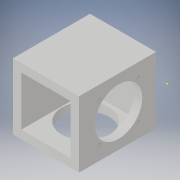
# Autodesk Inventor part: chamber
Saved by Autodesk Inventor 2019 (Build 230136000, 136)
## iProperties
Created: 2019-01-15
Part Number: chamber
Material: Generic
Document SubType Name: Sheet Metal
Designer: voras
Density: 1 g/cm^3
Appearance: Default
Sheet Metal Rule: Default
Author: voras
Autodesk Inventor part; units mm, degrees
ref_plane "YZ Plane" through (0, 0, 0) normal (1, 0, 0) x (0, 1, 0)
ref_plane "XZ Plane" through (0, 0, 0) normal (0, 1, 0) x (-1, 0, 0)
ref_plane "XY Plane" through (0, 0, 0) normal (0, 0, 1) x (1, 0, 0)
sketch "Sketch1" plane through (0, 0, 0) normal (0, 0, 1) x (1, 0, 0)
  point P0 (0, 0)
sketch "Sketch2" plane through (0, 0, 0) normal (0, 0, 1) x (1, 0, 0)
  line L0 (-22.5, 22.5) -> (22.5, 22.5)
  line L1 (22.5, 22.5) -> (22.5, -22.5)
  line L2 (22.5, -22.5) -> (-22.5, -22.5)
  line L3 (-22.5, -22.5) -> (-22.5, 22.5)
  line L4 (-22.5, 22.5) -> (22.5, -22.5) construction
  line L5 (22.5, 22.5) -> (-22.5, -22.5) construction
  line L6 (30, -30) -> (-30, -30)
  line L7 (-30, -30) -> (-30, 30)
  line L8 (-30, 30) -> (30, 30)
  line L9 (30, 30) -> (30, -30)
  line L10 (30, -30) -> (-30, 30) construction
  line L11 (-30, -30) -> (30, 30) construction
  point P0 (0, 0)
  dimension "d0" = 45
  dimension "d1" = 45
  dimension "d2" = 60
  dimension "d3" = 60
  constraints: 24 end point, 4 midpoint, 4 parallel, 2 horizontal, 2 perpendicular
  measures "d0" distance of L1.end L2.end
  measures "d1" distance of L0.end L1.end
  measures "d2" distance of L7.end L8.end
  measures "d3" distance of L6.end L7.end
extrude "Extrusion1" add sketch "Sketch2" along normal blind 55
sketch "Sketch3" plane through (0, 0, 0) normal (0, 0, 1) x (1, 0, 0)
  line L0 (-22.5, 22.5) -> (22.5, 22.5) projected
  line L1 (22.5, 22.5) -> (22.5, -22.5) projected
  line L2 (-22.5, 22.5) -> (22.5, 22.5)
  line L3 (22.5, 22.5) -> (22.5, -22.5)
  line L4 (22.5, -22.5) -> (-22.5, -22.5)
  line L5 (-22.5, -22.5) -> (-22.5, 22.5)
  point P0 (0, 0)
  constraints: 8 end point, 2 parallel, 1 horizontal, 1 perpendicular
extrude "Extrusion2" add sketch "Sketch3" along normal blind 20
sketch "Sketch6" plane through (30, -38.0357, 69.5741) normal (1, 0, 0) x (0, 0, -1)
  circle A0 centre (25.5741, 38.0357) radius 21.5
  line L0 (69.5741, 8.0357) -> (14.5741, 8.0357) projected
  line L1 (14.5741, 8.0357) -> (14.5741, 68.0357) projected
  point P0 (30, 0)
  dimension "d36" = 43
  dimension "d37" = 30
  dimension "d38" = 11
  constraints: 1 centre point
  measures "d36" diameter of A0
  measures "d37" distance from line of L0 A0.centre
  measures "d38" distance from line of A0.centre L1
extrude "Extrusion5" cut sketch "Sketch6" against normal blind 20
sketch "Sketch5" plane through (-30, -30, 0) normal (0, -1, 0) x (1, 0, 0)
  circle A0 centre (30, 44) radius 21.5
  line L0 (0, 0) -> (0, 55) projected
  line L1 (0, 55) -> (60, 55) projected
  point P0 (30, 0)
  dimension "d33" = 43
  dimension "d34" = 30
  dimension "d35" = 11
  constraints: 1 centre point
  measures "d33" diameter of A0
  measures "d34" distance from line of L0 A0.centre
  measures "d35" distance from line of L1 A0.centre
extrude "Extrusion4" cut sketch "Sketch5" against normal blind 20
fillet "Fillet3" radius 1 4 edges at (-22.5, 0, 20) (0, -22.5, 20) (22.5, 0, 20) (0, 22.5, 20)
sketch "Sketch9" plane through (30, -30, 0) normal (1, 0, 0) x (0, 0, -1)
  point P0 (0, 30)
move faces "Move Face1" translate (0, 0, 25) faces at (-27.5, -7.5, 55) (23.6577, -27.5, 55)
move faces "Move Face2" translate (0, 0, 10) faces at (10, 10, 0)
sketch "Sketch10" plane through (-30.0536, -30, 10.5547) normal (0, -1, 0) x (1, 0, 0)
  circle A0 centre (12.323, 15.843) radius 2.5
  circle A1 centre (30, 33.52) radius 21.5
  circle A2 centre (47.677, 15.843) radius 2.5
  circle A3 centre (47.677, 51.197) radius 2.5
  circle A4 centre (12.323, 51.197) radius 2.5
  point P0 (0, 0)
  dimension "d62" = 5
  dimension "d64" = 17.677
  dimension "d63" = 17.677
  dimension "d61" = 360
  constraints: 5 centre point, 9 other
  measures "d62" diameter of A0
  measures "d64" horizontal distance of A1.centre A0.centre
  measures "d63" horizontal distance of A1.centre A0.centre
hole "Hole3" at (17.6234, -30, 26.3977) at (-17.7306, -30, 26.3977) at (-17.7306, -30, 61.7517) at (17.6234, -30, 61.7517) direction (0, 1, 0) diameter 3.302 depth 4 thread size "8-32 UNC" class "2B" standard "ANSI Unified Screw Threads"
sketch "Sketch11" plane through (30, -33.5311, 74.1445) normal (1, 0, 0) x (0, 0, -1)
  circle A0 centre (12.323, 15.843) radius 2.5
  circle A1 centre (30, 33.52) radius 21.5
  circle A2 centre (47.677, 15.843) radius 2.5
  circle A3 centre (47.677, 51.197) radius 2.5
  circle A4 centre (12.323, 51.197) radius 2.5
  point P0 (0, 0)
  dimension "d75" = 5
  dimension "d77" = 17.677
  dimension "d76" = 17.677
  dimension "d74" = 360
  constraints: 5 centre point, 9 other
  measures "d75" diameter of A0
  measures "d77" horizontal distance of A1.centre A0.centre
  measures "d76" horizontal distance of A1.centre A0.centre
hole "Hole4" at (30, -17.6881, 26.4675) at (30, -17.6881, 61.8215) at (30, 17.6659, 61.8215) at (30, 17.6659, 26.4675) direction (-1, 0, 0) diameter 3.302 depth 4 thread size "8-32 UNC" class "2B" standard "ANSI Unified Screw Threads"
sketch "Sketch12" plane through (-33.4623, -33.3136, 10) normal (0, 0, -1) x (-1, 0, 0)
  circle A0 centre (-33.52, 33.52) radius 4.2426
  line L0 (0, 0) -> (-67.04, 0)
  line L1 (-67.04, 0) -> (-67.04, 67.04)
  dimension "d86" = 33.52
  dimension "d93" = 67.04
  dimension "d85" = 33.52
  dimension "d94" = 67.04
  constraints: 4 end point, 1 centre point
  measures "d86" distance from line of L0 A0.centre
  measures "d93" distance of L0.start L0.end
  measures "d85" distance from line of L1 A0.centre
  measures "d94" distance of L0.end L1.end
hole "Hole5" at (0.0577, 0.2064, 10) direction (0, 0, 1) diameter 4.978 depth 4
equation "\"d86\" = 0.5 * d93"
equation "\"d85\" = 0.5 * d94"
equation "\"BendRadius\" = Thickness"
equation "\"BendReliefWidth\" = Thickness"
equation "\"BendReliefDepth\" = 0.5 * Thickness"
equation "\"CornerReliefSize\" = 4 * Thickness"
equation "\"MinimumRemnant\" = 2 * Thickness"
equation "\"TransitionRadius\" = BendRadius"
equation "\"JacobiRadiusSize\" = Thickness"
equation "\"GapSize\" = Thickness"
equation "\"d131\" = Thickness"
equation "\"d158\" = Thickness"
equation "\"d179\" = Thickness"
equation "\"Thickness\" = 0.5"
body "Solid1"
